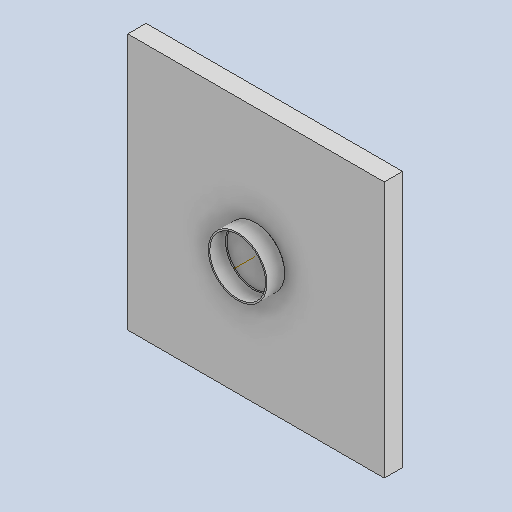
# Autodesk Inventor part: крепеж доска+доска
Saved by Autodesk Inventor 2023 (Build 270158000, 158)
## iProperties
Created: 2024-01-16
Part Number: крепеж доска+доска
Material: Типовые
Document SubType Name: Modeling
Designer: liza
Density: 1 g/cm^3
Appearance: По умолчанию
Author: liza
Autodesk Inventor part; units mm, degrees
ref_plane "YZ Plane" through (0, 0, 0) normal (1, 0, 0) x (0, 1, 0)
ref_plane "XZ Plane" through (0, 0, 0) normal (0, 1, 0) x (-1, 0, 0)
ref_plane "XY Plane" through (0, 0, 0) normal (0, 0, 1) x (1, 0, 0)
sketch "Эскиз3" plane through (0, 0, 0) normal (0, 1, 0) x (-1, 0, 0)
  line L0 (0, 0) -> (-78, 0)
  arc A0 (-80, 2) -> (-78, 0) centre (-78, 2) ccw
  line L1 (-2.0712, 5) -> (-74, 5)
  arc A1 (-76, 7) -> (-74, 5) centre (-74, 7) ccw
  line L2 (0, 0) -> (0, 5)
  line L3 (0, 5) -> (-2.0712, 5)
  line L4 (0, -10.4971) -> (0, 60.0828) projected
  line L5 (-80, 2) -> (-80, 50)
  line L6 (-76, 7) -> (-76, 50)
  line L7 (-76, 50) -> (-80, 50)
  dimension "d7" = 5
  dimension "d11" = 48
  constraints: 14 end point, 4 point on circle, 3 vertical, 2 centre point, 1 collinear, 1 perpendicular, 1 point on line, 1 tangent
  measures "d7" distance of L0.start L2.end
  measures "d11" distance of L5.start L5.end
revolve "Вращение1" add sketch "Эскиз3" angle 360 about axis through (0, 0, -10) along (0, 0, 1)
sketch "Эскиз4" plane through (0, 0, 0) normal (0, 0, -1) x (-1, 0, 0)
  point P0 (0, 0)
sketch "Эскиз5" plane through (0, 0, 0) normal (0, 0, -1) x (-1, 0, 0)
  line L0 (350, -350) -> (-350, -350)
  line L1 (-350, -350) -> (-350, 350)
  line L2 (-350, 350) -> (350, 350)
  line L3 (350, 350) -> (350, -350)
  line L4 (350, -350) -> (-350, 350) construction
  line L5 (-350, -350) -> (350, 350) construction
  point P0 (0, 0)
  dimension "d12" = 700
  dimension "d13" = 700
  constraints: 12 end point, 2 midpoint, 2 parallel, 1 horizontal, 1 perpendicular
  measures "d12" distance of L1.end L2.end
  measures "d13" distance of L0.end L1.end
extrude "Выдавливание2" add sketch "Эскиз5" along normal blind 50 separate body
